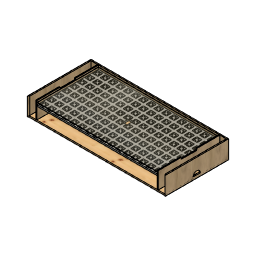
Built+to+size (Autodesk Fusion 360 design; units mm, degrees)
Autodesk Fusion 360 part; units mm, degrees
note: some values were not read from the file. Chosen so that the rebuilt part matches the saved one: a direction.
sketch "Sketch1" plane through (0, 0, 0) normal (0, 1, 0) x (1, 0, 0)
  line L0 (0, 0) -> (15.875, 0)
  line L1 (15.875, 0) -> (15.875, -844.55)
  line L2 (15.875, -844.55) -> (0, -844.55)
  line L3 (0, -844.55) -> (0, 0)
  dimension "d1" = 15.875
  dimension "d2" = 844.55
  constraint horizontal L0
  constraint vertical L1
  constraint horizontal L2
  constraint vertical L3
  constraint coincident L0.start L3.end
  measures "d1" distance of L0.start L0.end
  measures "d2" distance of L0.start L2.end
extrude "Extrude1" add sketch "Sketch1" along normal blind 241.3 makes body 1 in component "outside short edge L"
sketch "Sketch2" plane through (15.875, 0, 0) normal (1, 0, 0) x (0, 0, -1)
  line L0 (-844.55, 0) -> (0, 0)
  line L1 (0, 0) -> (0, 241.3)
  line L2 (0, 241.3) -> (-844.55, 241.3)
  line L3 (-844.55, 241.3) -> (-844.55, 0)
  line L4 (0, 0) -> (0, 18.2563)
  line L5 (0, 18.2563) -> (-844.55, 18.2563)
  dimension "d5" = 18.2563
  dimension "d6" = 844.55
  constraint coincident L0.end L1.start
  constraint perpendicular L0 L4
  constraint perpendicular L1 L5
  measures "d5" distance of L0.end L4.end
  measures "d6" distance of L4.end L5.end
extrude "Extrude2" cut sketch "Sketch2" against normal blind 6.35 contours L0 L1 L3 L4 L5 bodies 1 in component "outside short edge L"
sketch "Sketch3" plane through (0, 241.3, 0) normal (0, 1, 0) x (-1, 0, 0)
  line L0 (0, 844.55) -> (-15.875, 844.55)
  line L1 (-15.875, 844.55) -> (-15.875, 0)
  line L2 (-15.875, 0) -> (0, 0)
  line L3 (0, 0) -> (0, 844.55)
  line L4 (0, 0) -> (-15.875, 15.875)
  line L5 (0, 0) -> (22.4506, 0) construction
  dimension "d9" = 135
  constraint horizontal L5
  constraint coincident L2.end L3.start
  constraint coincident L1 L4.end
  measures "d9" angle of L4 L5
extrude "Extrude3" cut sketch "Sketch3" against normal blind 1270 contours L1 L2 L4 bodies 1 in component "outside short edge L"
sketch "Sketch4" plane through (0, 241.3, 0) normal (0, 1, 0) x (-1, 0, 0)
  line L0 (-15.875, 15.875) -> (0, 0)
  line L1 (0, 0) -> (0, 844.55)
  line L2 (0, 844.55) -> (-15.875, 844.55)
  line L3 (-15.875, 844.55) -> (-15.875, 15.875)
  line L4 (0, 844.55) -> (-15.875, 828.675)
  line L5 (0, 844.55) -> (22.4506, 844.55) construction
  dimension "d12" = 135
  constraint horizontal L5
  constraint coincident L1.end L2.start
  constraint coincident L3 L4.end
  measures "d12" angle of L4 L5
extrude "Extrude4" cut sketch "Sketch4" against normal blind 1270 contours L2 L3 L4 bodies 1 in component "outside short edge L"
sketch "Sketch5" plane through (0, 0, 0) normal (0, 1, 0) x (1, 0, 0)
  line L0 (0, 0) -> (1828.8, 0)
  line L1 (1828.8, 0) -> (1828.8, -15.875)
  line L2 (1828.8, -15.875) -> (0, -15.875)
  line L3 (0, -15.875) -> (0, 0)
  dimension "d15" = 1828.8
  dimension "d16" = 15.875
  constraint horizontal L0
  constraint vertical L1
  constraint horizontal L2
  constraint vertical L3
  constraint coincident L0.start L3.end
  measures "d15" distance of L0.start L0.end
  measures "d16" distance of L0.start L2.end
extrude "Extrude1'" add sketch "Sketch5" along normal blind 241.3 separate body makes body 2 in component "outside long edge U"
sketch "Sketch6" plane through (0, 0, 15.875) normal (0, 0, 1) x (1, 0, 0)
  line L0 (0, 0) -> (1828.8, 0)
  line L1 (1828.8, 0) -> (1828.8, 241.3)
  line L2 (1828.8, 241.3) -> (0, 241.3)
  line L3 (0, 241.3) -> (0, 0)
  line L4 (0, 0) -> (0, 18.2562)
  line L5 (0, 18.2562) -> (1828.8, 18.2562)
  dimension "d19" = 18.2563
  dimension "d20" = 1828.8
  constraint coincident L0.start L3.end
  constraint perpendicular L0 L4
  constraint perpendicular L3 L5
  measures "d19" distance of L0.start L4.end
  measures "d20" distance of L4.end L5.end
extrude "Extrude2'" cut sketch "Sketch6" against normal blind 6.35 contours L0 L1 L3 L4 L5 bodies 2 in component "outside long edge U"
sketch "Sketch7" plane through (0, 241.3, 0) normal (0, 1, 0) x (-1, 0, 0)
  line L0 (0, 15.875) -> (-1828.8, 15.875)
  line L1 (-1828.8, 15.875) -> (-1828.8, 0)
  line L2 (-1828.8, 0) -> (0, 0)
  line L3 (0, 0) -> (0, 15.875)
  line L4 (0, 0) -> (-15.875, 15.875)
  line L5 (0, 0) -> (22.4506, 0) construction
  dimension "d23" = 135
  constraint horizontal L5
  constraint coincident L2.end L3.start
  constraint coincident L0 L4.end
  measures "d23" angle of L4 L5
extrude "Extrude3'" cut sketch "Sketch7" against normal blind 1270 contours L0 L3 L4 bodies 2 in component "outside long edge U"
sketch "Sketch8" plane through (0, 241.3, 0) normal (0, 1, 0) x (-1, 0, 0)
  line L0 (0, 0) -> (-15.875, 15.875)
  line L1 (-15.875, 15.875) -> (-1828.8, 15.875)
  line L2 (-1828.8, 15.875) -> (-1828.8, 0)
  line L3 (-1828.8, 0) -> (0, 0)
  line L4 (-1828.8, 0) -> (-1812.925, 15.875)
  line L5 (-1828.8, 0) -> (-1806.3494, 0) construction
  dimension "d26" = 45
  constraint horizontal L5
  constraint coincident L2.end L3.start
  constraint coincident L1 L4.end
  measures "d26" angle of L4 L5
extrude "Extrude4'" cut sketch "Sketch8" against normal blind 254 contours L1 L2 L4 bodies 2 in component "outside long edge U"
sketch "Sketch9" plane through (0, 0, 0) normal (0, 1, 0) x (1, 0, 0)
  line L0 (0, 0) -> (0, -9.525)
  line L1 (0, -9.525) -> (9.525, -9.525)
  line L2 (9.525, -9.525) -> (1819.275, -9.525)
  line L3 (1819.275, -9.525) -> (1819.275, -835.025)
  line L4 (1819.275, -835.025) -> (9.525, -835.025)
  line L5 (9.525, -835.025) -> (9.525, -9.525)
  dimension "d29" = 9.525
  dimension "d30" = 9.525
  dimension "d31" = 1809.75
  dimension "d32" = 825.5
  constraint coincident L0.start origin
  constraint vertical L0
  constraint perpendicular L0 L1
  constraint horizontal L2
  constraint vertical L3
  constraint horizontal L4
  constraint vertical L5
  measures "d29" distance of L0.start L0.end
  measures "d30" distance of L0.end L1.end
  measures "d31" distance of L1.end L2.end
  measures "d32" distance of L1.end L4.end
extrude "Extrude1''" add sketch "Sketch9" along normal blind 18.2563 separate body makes body 3 in component "plywood base"
ref_plane "WorkPlane1" through (914.4, 9.1281, 422.275) normal (-1, 0, 0) x (0, 0, 1)
ref_plane "WorkPlane2" through (914.4, 9.1281, 422.275) normal (0, 0, 1) x (1, 0, 0)
mirror "MirrorComponent1" about plane through (0, 0, 0) normal (0, 0, 1) of bodies 1 makes body 4 in component "outside short edge R"
sketch "Sketch10" plane through (0, 0, 15.875) normal (0, 0, 1) x (1, 0, 0)
  line L0 (1812.925, 18.2562) -> (1812.925, 241.3)
  line L1 (1812.925, 241.3) -> (15.875, 241.3)
  line L2 (15.875, 241.3) -> (15.875, 18.2562)
  line L3 (15.875, 18.2562) -> (1812.925, 18.2562)
  line L4 (15.875, 241.3) -> (101.6, 241.3)
  line L5 (101.6, 241.3) -> (114.3, 241.3)
  line L6 (114.3, 241.3) -> (1714.5, 241.3)
  line L7 (1714.5, 241.3) -> (1727.2, 241.3)
  line L8 (1727.2, 241.3) -> (1812.925, 241.3)
  line L9 (101.6, 241.3) -> (101.6, 18.2562)
  line L10 (101.6, 18.2562) -> (114.3, 18.2562)
  line L11 (114.3, 18.2562) -> (114.3, 241.3)
  line L12 (114.3, 241.3) -> (101.6, 241.3)
  line L13 (101.6, 241.3) -> (101.6, 18.2562)
  line L14 (1727.2, 241.3) -> (1727.2, 18.2562)
  line L15 (1714.5, 241.3) -> (1727.2, 241.3)
  line L16 (1727.2, 241.3) -> (1727.2, 18.2562)
  line L17 (1727.2, 18.2562) -> (1714.5, 18.2562)
  line L18 (1714.5, 18.2562) -> (1714.5, 241.3)
  dimension "d35" = 85.725
  dimension "d36" = 12.7
  dimension "d37" = 1600.2
  dimension "d38" = 12.7
  constraint coincident L1.end L2.start
  constraint perpendicular L2 L4
  constraint parallel L1 L5
  constraint parallel L1 L6
  constraint parallel L1 L7
  constraint coincident L0.end L1.start
  constraint coincident L3 L9.end
  constraint perpendicular L3 L9
  constraint horizontal L10
  constraint vertical L11
  constraint horizontal L12
  constraint vertical L13
  constraint coincident L3 L14.end
  constraint perpendicular L3 L14
  constraint horizontal L15
  constraint vertical L16
  constraint horizontal L17
  constraint vertical L18
  measures "d35" distance of L1.end L4.end
  measures "d36" distance of L4.end L5.end
  measures "d37" distance of L5.end L6.end
  measures "d38" distance of L6.end L7.end
extrude "Extrude5" cut sketch "Sketch10" against normal blind 4.7625 contours L1 L3 L7 L14 L15 L16 L17 L18 bodies 2 in component "outside long edge U"
mirror "Mirror1" about plane through (914.4, 9.1281, 422.275) normal (-1, 0, 0) of "Extrude5" in component "outside long edge U"
mirror "MirrorComponent2" about plane through (0, 0, 0) normal (0, 0, 1) of bodies 2 makes body 5 in component "outside long edge D"
sketch "Sketch11" plane through (0, 18.2563, 0) normal (0, 1, 0) x (-1, 0, 0)
  line L0 (-9.525, 835.025) -> (-1819.275, 835.025)
  line L1 (-1819.275, 835.025) -> (-1819.275, 9.525)
  line L2 (-1819.275, 9.525) -> (-9.525, 9.525)
  line L3 (-9.525, 9.525) -> (-9.525, 835.025)
sketch "Sketch12" plane through (0, 241.3, 0) normal (0, 1, 0) x (-1, 0, 0)
  line L0 (-114.3, 11.1125) -> (-114.3, 15.875)
  line L1 (-114.3, 15.875) -> (-1714.5, 15.875)
  line L2 (-1714.5, 15.875) -> (-1714.5, 11.1125)
  line L3 (-1714.5, 11.1125) -> (-1727.2, 11.1125)
  line L4 (-1727.2, 11.1125) -> (-1727.2, 15.875)
  line L5 (-1727.2, 15.875) -> (-1812.925, 15.875)
  line L6 (-1812.925, 15.875) -> (-1828.8, 0)
  line L7 (-1828.8, 0) -> (0, 0)
  line L8 (0, 0) -> (-15.875, 15.875)
  line L9 (-15.875, 15.875) -> (-101.6, 15.875)
  line L10 (-101.6, 15.875) -> (-101.6, 11.1125)
  line L11 (-101.6, 11.1125) -> (-114.3, 11.1125)
sketch "Sketch13" plane through (914.4, 241.3, 7.9375) normal (0, 1, 0) x (-1, 0, 0)
  line L0 (812.8, 3.175) -> (800.1, 3.175)
  line L1 (800.1, 3.175) -> (800.1, 825.5)
  line L2 (800.1, 825.5) -> (812.8, 825.5)
  line L3 (812.8, 825.5) -> (812.8, 3.175)
  constraint horizontal L0
  constraint vertical L1
  constraint horizontal L2
  constraint vertical L3
extrude "Extrude1'''" add sketch "Sketch13" against normal blind 222.25 separate body makes body 6 in component "inside short edge L"
mirror "MirrorComponent3" about plane through (0, 0, 0) normal (0, 0, 1) of bodies 6 makes body 7 in component "inside short edge R"
sketch "Sketch14" plane through (114.3, 0, 0) normal (1, 0, 0) x (0, 0, -1)
  line L0 (-11.1125, 240.5063) -> (-833.4375, 240.5063)
  line L1 (-833.4375, 240.5063) -> (-833.4375, 18.2563)
  line L2 (-833.4375, 18.2563) -> (-11.1125, 18.2563)
  line L3 (-11.1125, 18.2563) -> (-11.1125, 240.5063)
sketch "Sketch15" plane through (0, 18.2563, 0) normal (0, 1, 0) x (-1, 0, 0)
sketch "Sketch16" plane through (0, 241.3, 0) normal (0, 1, 0) x (-1, 0, 0)
  line L0 (-114.3, 828.675) -> (-114.3, 833.4375)
  line L1 (-114.3, 833.4375) -> (-101.6, 833.4375)
  line L2 (-101.6, 833.4375) -> (-101.6, 828.675)
  line L3 (-101.6, 828.675) -> (-15.875, 828.675)
  line L4 (-15.875, 828.675) -> (0, 844.55)
  line L5 (0, 844.55) -> (-1828.8, 844.55)
  line L6 (-1828.8, 844.55) -> (-1812.925, 828.675)
  line L7 (-1812.925, 828.675) -> (-1727.2, 828.675)
  line L8 (-1727.2, 828.675) -> (-1727.2, 833.4375)
  line L9 (-1727.2, 833.4375) -> (-1714.5, 833.4375)
  line L10 (-1714.5, 833.4375) -> (-1714.5, 828.675)
  line L11 (-1714.5, 828.675) -> (-114.3, 828.675)
  line L12 (-1714.5, 828.675) -> (-114.3, 828.675)
  line L13 (-114.3, 828.675) -> (-114.3, 15.875)
  line L14 (-114.3, 15.875) -> (-1714.5, 15.875)
  line L15 (-1714.5, 15.875) -> (-1714.5, 828.675)
  dimension "d45" = 1600.2
  dimension "d46" = 812.8
  constraint horizontal L12
  constraint vertical L13
  constraint horizontal L14
  constraint vertical L15
  constraint coincident L10.end L11.start
  measures "d45" distance of L10.end L0.start
  measures "d46" distance of L10.end L14.end
extrude "Extrude1''''" add sketch "Sketch16" against normal blind 19.05 separate body contours L11 L12 L13 L14 L15 makes body 8 in component "mdf"
sketch "Sketch17" plane through (0, 241.3, 0) normal (0, 1, 0) x (-1, 0, 0)
  line L0 (-1714.5, 15.875) -> (-114.3, 15.875)
  line L1 (-114.3, 15.875) -> (-114.3, 828.675)
  line L2 (-114.3, 828.675) -> (-1714.5, 828.675)
  line L3 (-1714.5, 828.675) -> (-1714.5, 15.875)
  line L4 (-1714.5, 828.675) -> (-114.3, 828.675)
  line L5 (-114.3, 828.675) -> (-114.3, 15.875)
  line L6 (-114.3, 15.875) -> (-1714.5, 15.875)
  line L7 (-1714.5, 15.875) -> (-1714.5, 828.675)
  constraint horizontal L4
  constraint vertical L5
  constraint horizontal L6
  constraint vertical L7
  constraint coincident L0.end L1.start
  constraint coincident L2.end L3.start
extrude "Extrude1'''''" add sketch "Sketch17" along normal blind 3.175 separate body makes body 9 in component "acrylic"
sketch "Sketch18" plane through (1714.5, 0, 0) normal (-1, 0, 0) x (0, 0, 1)
  line L0 (833.4375, 240.5062) -> (11.1125, 240.5062)
  line L1 (11.1125, 240.5062) -> (11.1125, 18.2562)
  line L2 (11.1125, 18.2562) -> (833.4375, 18.2562)
  line L3 (833.4375, 18.2562) -> (833.4375, 240.5062)
sketch "Sketch19" plane through (114.3, 0, 0) normal (1, 0, 0) x (0, 0, -1)
sketch "Sketch20" plane through (1714.5, 129.3812, 422.275) normal (-1, 0, 0) x (0, 0, 1)
  line L0 (0, 111.125) -> (-101.6, 111.125)
  line L1 (-101.6, 111.125) -> (101.6, 111.125)
  line L2 (101.6, 111.125) -> (101.6, 88.9)
  line L3 (101.6, 88.9) -> (-101.6, 88.9)
  line L4 (-101.6, 88.9) -> (-101.6, 111.125)
  dimension "d51" = 101.6
  dimension "d52" = 203.2
  dimension "d53" = 22.225
  constraint horizontal L1
  constraint vertical L2
  constraint horizontal L3
  constraint vertical L4
  measures "d51" distance of L0.start L0.end
  measures "d52" distance of L0.end L1.end
  measures "d53" distance of L0.end L3.end
extrude "Extrude1''''''" cut sketch "Sketch20" against normal blind 101.6 sketch seen with x (-1, 0, 0) y (0, 1, 0) z (0, 0, -1) at (1828.8, 0.7938, 0) bodies 7 in component "inside short edge R"
sketch "Sketch21" plane through (101.6, 0, 0) normal (-1, 0, 0) x (0, 0, 1)
  line L0 (833.4375, 240.5062) -> (11.1125, 240.5062)
  line L1 (11.1125, 240.5062) -> (11.1125, 18.2562)
  line L2 (11.1125, 18.2562) -> (833.4375, 18.2562)
  line L3 (833.4375, 18.2562) -> (833.4375, 240.5062)
  line L4 (11.1125, 240.5062) -> (320.675, 240.5062)
  line L5 (320.675, 240.5062) -> (523.875, 240.5062)
  line L6 (523.875, 240.5062) -> (523.875, 218.2812)
  line L7 (523.875, 218.2812) -> (320.675, 218.2812)
  line L8 (320.675, 218.2812) -> (320.675, 240.5062)
  dimension "d56" = 309.5625
  dimension "d57" = 203.2
  dimension "d58" = 22.225
  constraint coincident L0.end L1.start
  constraint perpendicular L1 L4
  constraint horizontal L5
  constraint vertical L6
  constraint horizontal L7
  constraint vertical L8
  measures "d56" distance of L0.end L4.end
  measures "d57" distance of L4.end L5.end
  measures "d58" distance of L4.end L7.end
extrude "Extrude2''" cut sketch "Sketch21" against normal blind 101.6 contours L0 L5 L6 L7 L8 sketch seen with x (1, 0, 0) y (0, 1, 0) z (0, 0, 1) at (0, 0.7938, 0) bodies 6 in component "inside short edge L"
sketch "Sketch22" plane through (0, 190.5, 0) normal (0, 1, 0) x (-1, 0, 0)
  line L0 (-1714.5, 15.875) -> (-114.3, 15.875)
  line L1 (-114.3, 15.875) -> (-114.3, 828.675)
  line L2 (-114.3, 828.675) -> (-1714.5, 828.675)
  line L3 (-1714.5, 828.675) -> (-1714.5, 15.875)
sketch "Sketch23" plane through (914.4, 190.5, 422.275) normal (0, 1, 0) x (-1, 0, 0)
  line L0 (0, 0) -> (0, -101.6)
  line L1 (0, -101.6) -> (0, -203.2)
  line L2 (0, -203.2) -> (0, -304.8)
  line L3 (0, -304.8) -> (0, -406.4)
  line L4 (0, 0) -> (-101.6, 0)
  line L5 (-101.6, 0) -> (-203.2, 0)
  line L6 (-203.2, 0) -> (-304.8, 0)
  line L7 (-304.8, 0) -> (-406.4, 0)
  line L8 (-406.4, 0) -> (-508, 0)
  line L9 (-508, 0) -> (-609.6, 0)
  line L10 (-609.6, 0) -> (-711.2, 0)
  line L11 (-711.2, 0) -> (-800.1, 0)
  line L12 (0, -101.6) -> (0, -82.55)
  line L13 (0, 0) -> (0, -19.05)
  line L14 (0, 0) -> (-19.05, 0)
  line L15 (-19.05, -19.05) -> (-86.36, -19.05)
  line L16 (-86.36, -19.05) -> (-86.36, -82.55)
  line L17 (-86.36, -82.55) -> (-19.05, -82.55)
  line L18 (-19.05, -82.55) -> (-19.05, -19.05)
  line L19 (-800.1, -406.4) -> (-797.56, -406.4)
  line L20 (-797.56, -406.4) -> (-797.56, -387.35)
  line L21 (-797.56, -387.35) -> (-730.25, -387.35)
  line L22 (-730.25, -387.35) -> (-730.25, -323.85)
  line L23 (-730.25, -323.85) -> (-797.56, -323.85)
  line L24 (-797.56, -323.85) -> (-797.56, -387.35)
  dimension "d61" = 101.6
  dimension "d62" = 101.6
  dimension "d63" = 101.6
  dimension "d64" = 101.6
  dimension "d65" = 101.6
  dimension "d66" = 101.6
  dimension "d67" = 101.6
  dimension "d68" = 101.6
  dimension "d69" = 101.6
  dimension "d70" = 101.6
  dimension "d71" = 101.6
  dimension "d72" = 88.9
  dimension "d73" = 19.05
  dimension "d74" = 19.05
  dimension "d75" = 19.05
  dimension "d76" = 67.31
  dimension "d77" = 63.5
  dimension "d78" = 2.54
  dimension "d79" = 19.05
  dimension "d80" = 67.31
  dimension "d81" = 63.5
  constraint coincident L0.start L4.start
  constraint vertical L0
  constraint parallel L0 L1
  constraint parallel L1 L2
  constraint parallel L2 L3
  constraint horizontal L4
  constraint parallel L4 L5
  constraint parallel L5 L6
  constraint parallel L6 L7
  constraint horizontal L8
  constraint parallel L8 L9
  constraint parallel L9 L10
  constraint parallel L10 L11
  constraint parallel L0 L12
  constraint perpendicular L4 L13
  constraint perpendicular L0 L14
  constraint horizontal L15
  constraint vertical L16
  constraint horizontal L17
  constraint vertical L18
  constraint horizontal L19
  constraint perpendicular L19 L20
  constraint horizontal L21
  constraint vertical L22
  constraint horizontal L23
  constraint vertical L24
  measures "d61" distance of L0.start L0.end
  measures "d62" distance of L0.end L1.end
  measures "d63" distance of L1.end L2.end
  measures "d64" distance of L2.end L3.end
  measures "d65" distance of L0.start L4.end
  measures "d66" distance of L4.end L5.end
  measures "d67" distance of L5.end L6.end
  measures "d68" distance of L6.end L7.end
  measures "d69" distance of L7.end L8.end
  measures "d70" distance of L8.end L9.end
  measures "d71" distance of L9.end L10.end
  measures "d72" distance of L10.end L11.end
  measures "d73" distance of L0.end L12.end
  measures "d74" distance of L0.start L13.end
  measures "d75" distance of L0.start L14.end
  measures "d76" distance of L15.start L15.end
  measures "d77" distance of L15.start L17.end
  measures "d78" distance of L19.start L19.end
  measures "d79" distance of L19.end L20.end
  measures "d80" distance of L20.end L21.end
  measures "d81" distance of L20.end L23.end
extrude "Extrude2'''" cut sketch "Sketch23" against normal blind 1.524 contours L21 L22 L23 L24 sketch seen with x (1, 0, 0) y (0, 1, 0) z (0, 0, 1) at (0, 50.8, 0) bodies 8 in component "mdf"
sketch "Sketch24" plane through (914.4, 190.5, 422.275) normal (0, 1, 0) x (-1, 0, 0)
  line L0 (-800.1, -406.4) -> (-797.56, -406.4)
  line L1 (-797.56, -406.4) -> (-797.56, -387.35)
  line L2 (-797.56, -387.35) -> (-730.25, -387.35)
  line L3 (-730.25, -387.35) -> (-730.25, -323.85)
  line L4 (-730.25, -323.85) -> (-797.56, -323.85)
  line L5 (-797.56, -323.85) -> (-797.56, -387.35)
  line L6 (-730.25, -387.35) -> (-730.25, -377.19)
  line L7 (-730.25, -377.19) -> (-797.56, -377.19)
  line L8 (-730.25, -377.19) -> (-730.25, -372.11)
  line L9 (-730.25, -372.11) -> (-797.56, -372.11)
  line L10 (-730.25, -323.85) -> (-730.25, -334.01)
  line L11 (-730.25, -334.01) -> (-797.56, -334.01)
  line L12 (-730.25, -334.01) -> (-730.25, -339.09)
  line L13 (-730.25, -339.09) -> (-797.56, -339.09)
  line L14 (-797.56, -387.35) -> (-787.4, -387.35)
  line L15 (-787.4, -387.35) -> (-787.4, -323.85)
  line L16 (-787.4, -387.35) -> (-782.32, -387.35)
  line L17 (-782.32, -387.35) -> (-782.32, -323.85)
  line L18 (-782.32, -387.35) -> (-744.22, -387.35)
  line L19 (-744.22, -387.35) -> (-744.22, -323.85)
  line L20 (-744.22, -323.85) -> (-739.14, -323.85)
  line L21 (-739.14, -323.85) -> (-739.14, -387.35)
  line L22 (-782.32, -387.35) -> (-767.08, -387.35)
  line L23 (-767.08, -387.35) -> (-756.92, -387.35)
  line L24 (-756.92, -387.35) -> (-756.92, -323.85)
  line L25 (-767.08, -387.35) -> (-767.08, -323.85)
  line L26 (-797.56, -339.09) -> (-797.56, -344.17)
  line L27 (-797.56, -344.17) -> (-730.25, -344.17)
  line L28 (-797.56, -344.17) -> (-797.56, -369.57)
  line L29 (-797.56, -369.57) -> (-730.25, -369.57)
  dimension "d84" = 2.54
  dimension "d85" = 19.05
  dimension "d86" = 67.31
  dimension "d87" = 63.5
  dimension "d88" = 10.16
  dimension "d89" = 67.31
  dimension "d90" = 5.08
  dimension "d91" = 10.16
  dimension "d92" = 5.08
  dimension "d93" = 10.16
  dimension "d94" = 5.08
  dimension "d95" = 38.1
  dimension "d96" = 5.08
  dimension "d97" = 15.24
  dimension "d98" = 10.16
  dimension "d99" = 5.08
  dimension "d100" = 25.4
  constraint horizontal L0
  constraint perpendicular L0 L1
  constraint horizontal L2
  constraint vertical L3
  constraint horizontal L4
  constraint vertical L5
  constraint perpendicular L2 L6
  constraint perpendicular L3 L7
  constraint perpendicular L7 L8
  constraint coincident L5 L9.end
  constraint perpendicular L5 L9
  constraint perpendicular L4 L10
  constraint coincident L5 L11.end
  constraint perpendicular L5 L11
  constraint perpendicular L11 L12
  constraint coincident L5 L13.end
  constraint perpendicular L5 L13
  constraint perpendicular L5 L14
  constraint coincident L4 L15.end
  constraint perpendicular L4 L15
  constraint perpendicular L15 L16
  constraint coincident L4 L17.end
  constraint perpendicular L4 L17
  constraint perpendicular L17 L18
  constraint coincident L4 L19.end
  constraint perpendicular L4 L19
  constraint perpendicular L19 L20
  constraint coincident L2 L21.end
  constraint perpendicular L2 L21
  constraint perpendicular L17 L22
  constraint parallel L2 L23
  constraint coincident L4 L24.end
  constraint perpendicular L4 L24
  constraint coincident L4 L25.end
  constraint perpendicular L4 L25
  constraint perpendicular L13 L26
  constraint coincident L3 L27.end
  constraint perpendicular L3 L27
  constraint perpendicular L27 L28
  constraint coincident L3 L29.end
  constraint perpendicular L3 L29
  measures "d84" distance of L0.start L0.end
  measures "d85" distance of L0.end L1.end
  measures "d86" distance of L1.end L2.end
  measures "d87" distance of L1.end L4.end
  measures "d88" distance of L2.end L6.end
  measures "d89" distance of L6.end L7.end
  measures "d90" distance of L6.end L8.end
  measures "d91" distance of L3.end L10.end
  measures "d92" distance of L10.end L12.end
  measures "d93" distance of L1.end L14.end
  measures "d94" distance of L14.end L16.end
  measures "d95" distance of L16.end L18.end
  measures "d96" distance of L19.end L20.end
  measures "d97" distance of L16.end L22.end
  measures "d98" distance of L22.end L23.end
  measures "d99" distance of L13.end L26.end
  measures "d100" distance of L26.end L28.end
extrude "Extrude3''" cut sketch "Sketch24" against normal blind 9.525 contours L7 L9 L24 L25 | L15 L17 L27 L29 | L19 L21 L27 L29 | L11 L13 L24 L25 sketch seen with x (1, 0, 0) y (0, 1, 0) z (0, 0, 1) at (0, 50.8, 0) bodies 8 in component "mdf"
pattern_linear "R-Pattern1" count 8 spacing 101.6 along (0, 0, 1) count 16 spacing 101.6 along (-1, 0, 0) of "Extrude2'''", "Extrude3''" in component "mdf"
sketch "Sketch25" plane through (914.4, 190.5, 422.275) normal (0, 1, 0) x (-1, 0, 0)
  line L0 (0, 0) -> (0, -40.64)
  line L1 (0, -40.64) -> (27.94, -40.64)
  line L2 (27.94, -40.64) -> (-27.94, -40.64)
  line L3 (-27.94, -40.64) -> (-27.94, 40.64)
  line L4 (-27.94, 40.64) -> (27.94, 40.64)
  line L5 (27.94, 40.64) -> (27.94, -40.64)
  dimension "d108" = 40.64
  dimension "d109" = 27.94
  dimension "d110" = 55.88
  dimension "d111" = 81.28
  constraint coincident L0.start origin
  constraint vertical L0
  constraint perpendicular L0 L1
  constraint horizontal L2
  constraint vertical L3
  constraint horizontal L4
  constraint vertical L5
  measures "d108" distance of L0.start L0.end
  measures "d109" distance of L0.end L1.end
  measures "d110" distance of L1.end L2.end
  measures "d111" distance of L1.end L4.end
extrude "Extrude4''" cut sketch "Sketch25" against normal blind 2540 sketch seen with x (1, 0, 0) y (0, 1, 0) z (0, 0, 1) at (0, 50.8, 0) bodies 8 in component "mdf"
sketch "Sketch26" plane through (15.875, 0, 0) normal (1, 0, 0) x (0, 0, -1)
  line L0 (-828.675, 241.3) -> (-828.675, 18.2562)
  line L1 (-828.675, 18.2562) -> (-15.875, 18.2562)
  line L2 (-15.875, 18.2562) -> (-15.875, 241.3)
  line L3 (-15.875, 241.3) -> (-828.675, 241.3)
  line L4 (-828.675, 241.3) -> (-422.275, 241.3)
  line L5 (-422.275, 18.2562) -> (-422.275, 241.3)
  line L6 (-422.275, 18.2562) -> (-422.275, 38.1)
  line L7 (-422.275, 38.1) -> (-469.9, 38.1)
  line L8 (-422.275, 38.1) -> (-422.275, 78.74)
  line L9 (-422.275, 38.1) -> (-374.65, 38.1)
  line L10 (-469.9, 38.1) -> (-374.65, 38.1)
  line L11 (-469.9, 38.1) -> (-374.65, 38.1)
  circle A0 centre (-422.275, 38.1) radius 47.625
  dimension "d115" = 47.625
  dimension "d116" = 40.64
  dimension "d117" = 47.625
  constraint coincident L0.start L3.end
  constraint midpoint L3 L4.end
  constraint midpoint L1 L5.start
  constraint coincident L5 L6.end
  constraint perpendicular L1 L6
  constraint perpendicular L5 L7
  constraint perpendicular L7 L8
  constraint perpendicular L6 L9
  constraint coincident L9.end A0
  constraint coincident L7.end A0
  measures "d115" distance of L6.end L7.end
  measures "d116" distance of L6.end L8.end
  measures "d117" distance of L6.end L9.end
extrude "Extrude5'" cut sketch "Sketch26" against normal blind 50.8 contours L5 L8 L9 L10 L11 A0 | L5 L7 L8 L10 L11 A0 bodies 1 in component "outside short edge L"
sketch "Sketch27" plane through (1812.925, 0, 0) normal (-1, 0, 0) x (0, 0, 1)
  line L0 (828.675, 18.2562) -> (828.675, 241.3)
  line L1 (828.675, 241.3) -> (15.875, 241.3)
  line L2 (15.875, 241.3) -> (15.875, 18.2562)
  line L3 (15.875, 18.2562) -> (828.675, 18.2562)
  line L4 (374.65, 38.1) -> (469.9, 38.1)
  circle A0 centre (422.275, 38.1) radius 47.625
  constraint horizontal L4
  constraint coincident L4.end A0
  constraint coincident L4.start A0
extrude "Extrude1'''''''" cut sketch "Sketch27" against normal blind 5080 contours L4 A0 sketch seen with x (-1, 0, 0) y (0, 1, 0) z (0, 0, -1) at (1828.8, 0, 0) bodies 4 in component "outside short edge R"
component "outside short edge L" placed x (1, 0, 0) y (0, 1, 0) z (0, 0, 1) at (0, 0, 0)
component "outside long edge U" placed x (1, 0, 0) y (0, 1, 0) z (0, 0, 1) at (0, 0, 0)
component "plywood base" placed x (1, 0, 0) y (0, 1, 0) z (0, 0, 1) at (0, 0, 0)
component "outside short edge R" placed x (-1, 0, 0) y (0, 1, 0) z (0, 0, -1) at (1828.8, 0, 0)
component "outside long edge D" placed x (1, 0, 0) y (0, 1, 0) z (0, 0, 1) at (0, 0, 844.55)
component "inside short edge L" placed x (1, 0, 0) y (0, 1, 0) z (0, 0, 1) at (0, -0.7938, 0)
component "inside short edge R" placed x (-1, 0, 0) y (0, 1, 0) z (0, 0, -1) at (1828.8, -0.7938, 0)
component "mdf" placed x (1, 0, 0) y (0, 1, 0) z (0, 0, 1) at (0, -50.8, 0)
component "acrylic" placed x (1, 0, 0) y (0, 1, 0) z (0, 0, 1) at (0, -25.4, 0)
equation "d1 = ( 5 / 8 ) * 1 in"
equation "d5 = ( 23 / 32 ) * 1 in"
equation "d16 = ( 5 / 8 ) * 1 in"
equation "d19 = ( 23 / 32 ) * 1 in"
equation "d29 = ( 3 / 8 ) * 1 in"
equation "d30 = ( 3 / 8 ) * 1 in"
equation "d33 = ( 23 / 32 ) * 1 in"
equation "d39 = ( -3 / 16 ) * 1 in"
equation "d101 = ( -3 / 8 ) * 1 in"
